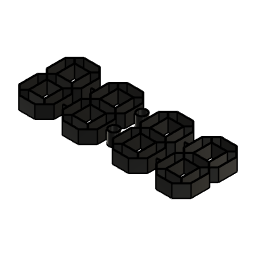
digitalclock_7segment_grid (Autodesk Fusion 360 design; units mm, degrees)
part number: Konfiguration 1
Autodesk Fusion 360 part; units mm, degrees
sketch "Skizze1" plane through (0, 0, 0) normal (0, 0, 1) x (1, 0, 0)
  line L0 (43.4571, -32.4142) -> (38.4571, -37.4142)
  line L1 (38.4571, -37.4142) -> (20.4571, -37.4142)
  line L2 (15.4571, -32.4142) -> (20.4571, -27.4142)
  line L3 (20.4571, -37.4142) -> (15.4571, -32.4142)
  line L4 (20.4571, -27.4142) -> (38.4571, -27.4142)
  line L5 (38.4571, -27.4142) -> (43.4571, -32.4142)
  line L6 (-92114.4293, 91329.2603) -> (-92111.6515, 91326.0366)
  line L7 (-92121.2848, 91323.3531) -> (-92114.4293, 91329.2603)
  line L8 (-92111.6515, 91326.0366) -> (-92106.8214, 91308.6967)
  line L9 (-92112.937, 91302.5267) -> (-92116.4546, 91306.0133)
  line L10 (-92116.4546, 91306.0133) -> (-92121.2848, 91323.3531)
  line L11 (-92118.8697, 91314.6832) -> (-92109.2364, 91317.3666) construction
  line L12 (-92106.8214, 91308.6967) -> (-92112.937, 91302.5267)
  line L13 (38.4571, -5) -> (20.4571, -5)
  line L14 (20.4571, 5) -> (38.4571, 5)
  line L15 (43.4571, 0) -> (38.4571, -5)
  line L16 (38.4571, 5) -> (43.4571, 0)
  line L17 (15.4571, 0) -> (20.4571, 5)
  line L18 (20.4571, -5) -> (15.4571, 0)
  line L19 (38.4571, 27.4142) -> (20.4571, 27.4142)
  line L20 (20.4571, 37.4142) -> (38.4571, 37.4142)
  line L21 (43.4571, 32.4142) -> (38.4571, 27.4142)
  line L22 (38.4571, 37.4142) -> (43.4571, 32.4142)
  line L23 (15.4571, 32.4142) -> (20.4571, 37.4142)
  line L24 (20.4571, 27.4142) -> (15.4571, 32.4142)
  line L25 (9.75, -26.7071) -> (9.75, -5.7071)
  line L26 (19.75, -5.7071) -> (19.75, -26.7071)
  line L27 (14.75, -31.7071) -> (9.75, -26.7071)
  line L28 (19.75, -26.7071) -> (14.75, -31.7071)
  line L29 (14.75, -0.7071) -> (19.75, -5.7071)
  line L30 (9.75, -5.7071) -> (14.75, -0.7071)
  line L31 (19.75, 5.7071) -> (14.75, 0.7071)
  line L32 (14.75, 0.7071) -> (9.75, 5.7071)
  line L33 (9.75, 26.7071) -> (14.75, 31.7071)
  line L34 (9.75, 5.7071) -> (9.75, 26.7071)
  line L35 (19.75, 26.7071) -> (19.75, 5.7071)
  line L36 (14.75, 31.7071) -> (19.75, 26.7071)
  line L37 (49.1642, -26.7071) -> (44.1642, -31.7071)
  line L38 (44.1642, -31.7071) -> (39.1642, -26.7071)
  line L39 (39.1642, -5.7071) -> (44.1642, -0.7071)
  line L40 (39.1642, -26.7071) -> (39.1642, -5.7071)
  line L41 (49.1642, -5.7071) -> (49.1642, -26.7071)
  line L42 (44.1642, -0.7071) -> (49.1642, -5.7071)
  line L43 (49.1642, 5.7071) -> (44.1642, 0.7071)
  line L44 (44.1642, 0.7071) -> (39.1642, 5.7071)
  line L45 (39.1642, 26.7071) -> (44.1642, 31.7071)
  line L46 (39.1642, 5.7071) -> (39.1642, 26.7071)
  line L47 (49.1642, 26.7071) -> (49.1642, 5.7071)
  line L48 (44.1642, 31.7071) -> (49.1642, 26.7071)
  line L49 (49.1642, -16.2071) -> (39.1642, -16.2071) construction
  line L50 (29.4571, -37.4142) -> (29.4571, -27.4142) construction
  line L51 (29.4571, -5) -> (29.4571, 5) construction
  line L52 (29.4571, 27.4142) -> (29.4571, 37.4142) construction
  line L53 (49.1642, 16.2071) -> (39.1642, 16.2071) construction
  line L54 (9.75, 16.2071) -> (19.75, 16.2071) construction
  line L55 (19.75, -16.2071) -> (9.75, -16.2071) construction
  line L56 (38.1642, -26.4142) -> (20.75, -26.4142)
  line L57 (20.75, -26.4142) -> (20.75, -6)
  line L58 (20.75, -6) -> (38.1642, -6)
  line L59 (38.1642, -6) -> (38.1642, -26.4142)
  line L60 (38.1642, 6) -> (20.75, 6)
  line L61 (20.75, 6) -> (20.75, 26.4142)
  line L62 (20.75, 26.4142) -> (38.1642, 26.4142)
  line L63 (38.1642, 26.4142) -> (38.1642, 6)
  line L64 (50.1642, 27.1213) -> (38.8713, 38.4142)
  line L65 (38.8713, 38.4142) -> (20.0429, 38.4142)
  line L66 (20.0429, 38.4142) -> (8.75, 27.1213)
  line L67 (8.75, -27.1213) -> (20.0429, -38.4142)
  line L68 (20.0429, -38.4142) -> (38.8713, -38.4142)
  line L69 (38.8713, -38.4142) -> (50.1642, -27.1213)
  line L70 (50.1642, 5.2929) -> (44.8713, 0)
  line L71 (44.8713, 0) -> (50.1642, -5.2929)
  line L72 (8.75, -5.2929) -> (14.0429, 0)
  line L73 (14.0429, 0) -> (8.75, 5.2929)
  line L74 (50.1642, -27.1213) -> (50.1642, -5.2929)
  line L75 (50.1642, 5.2929) -> (50.1642, 27.1213)
  line L76 (8.75, 27.1213) -> (8.75, 5.2929)
  line L77 (8.75, -5.2929) -> (8.75, -27.1213)
  line L78 (1.75, 0) -> (22.5, 0)
  dimension "d8" = 18
  dimension "d9" = 10
  dimension "d10" = 18
  dimension "d24" = 18
  dimension "d25" = 10
  dimension "d26" = 18
  dimension "d33" = 5
  dimension "d34" = 5
  dimension "d35" = 18
  dimension "d36" = 10
  dimension "d37" = 18
  dimension "d38" = 5
  dimension "d39" = 5
  dimension "d40" = 18
  dimension "d41" = 10
  dimension "d42" = 18
  dimension "d43" = 5
  dimension "d44" = 5
  dimension "d45" = 21
  dimension "d46" = 10
  dimension "d47" = 21
  dimension "d48" = 5
  dimension "d49" = 5
  dimension "d50" = 21
  dimension "d51" = 10
  dimension "d52" = 21
  dimension "d53" = 5
  dimension "d54" = 5
  dimension "d55" = 21
  dimension "d56" = 10
  dimension "d57" = 21
  dimension "d58" = 5
  dimension "d59" = 5
  dimension "d60" = 21
  dimension "d61" = 10
  dimension "d62" = 21
  dimension "d63" = 5
  dimension "d64" = 5
  dimension "d65" = 1
  dimension "d66" = 1
  dimension "d68" = 1
  dimension "d69" = 1
  dimension "d70" = 1
  dimension "d71" = 1
  dimension "d72" = 1
  dimension "d73" = 1
  dimension "d74" = 1
  dimension "d75" = 1
  dimension "d76" = 1
  dimension "d77" = 1
  dimension "d78" = 1
  dimension "d79" = 1
  dimension "d80" = 1
  dimension "d81" = 1
  dimension "d82" = 1
  dimension "d83" = 1
  dimension "d84" = 1
  dimension "d85" = 1
  dimension "d86" = 1
  dimension "d87" = 1
  dimension "d88" = 1
  dimension "d89" = 1
  dimension "d90" = 8.75
  constraint horizontal L1
  constraint perpendicular L2 L3
  constraint parallel L1 L4
  constraint perpendicular L0 L5
  constraint perpendicular L6 L7
  constraint parallel L8 L10
  constraint perpendicular L9 L12
  constraint midpoint L11.start L10
  constraint midpoint L11.end L8
  constraint perpendicular L10 L11
  constraint horizontal L13
  constraint perpendicular L17 L18
  constraint parallel L13 L14
  constraint perpendicular L15 L16
  constraint horizontal L19
  constraint perpendicular L23 L24
  constraint parallel L19 L20
  constraint perpendicular L21 L22
  constraint perpendicular L29 L30
  constraint parallel L25 L26
  constraint perpendicular L27 L28
  constraint perpendicular L33 L36
  constraint parallel L34 L35
  constraint perpendicular L31 L32
  constraint perpendicular L39 L42
  constraint parallel L40 L41
  constraint perpendicular L37 L38
  constraint perpendicular L45 L48
  constraint parallel L46 L47
  constraint perpendicular L43 L44
  constraint vertical L41
  constraint midpoint L41 L49.start
  constraint midpoint L40 L49.end
  constraint midpoint L1 L50.start
  constraint midpoint L4 L50.end
  constraint midpoint L13 L51.start
  constraint midpoint L14 L51.end
  constraint midpoint L19 L52.start
  constraint midpoint L20 L52.end
  constraint midpoint L47 L53.start
  constraint midpoint L46 L53.end
  constraint midpoint L34 L54.start
  constraint midpoint L35 L54.end
  constraint perpendicular L35 L54
  constraint midpoint L26 L55.start
  constraint midpoint L25 L55.end
  constraint perpendicular L25 L55
  constraint perpendicular L40 L49
  constraint perpendicular L1 L50
  constraint perpendicular L19 L52
  constraint perpendicular L13 L51
  constraint perpendicular L47 L53
  constraint collinear L0 L37
  constraint collinear L16 L42
  constraint collinear L17 L30
  constraint collinear L3 L27
  constraint collinear L15 L43
  constraint collinear L22 L48
  constraint collinear L18 L32
  constraint collinear L23 L33
  constraint horizontal L56
  constraint vertical L57
  constraint horizontal L58
  constraint vertical L59
  constraint horizontal L60
  constraint vertical L61
  constraint horizontal L62
  constraint vertical L63
  constraint perpendicular L37 L64
  constraint parallel L37 L66
  constraint parallel L41 L76
  constraint vertical L74
  constraint horizontal L68
  constraint horizontal L65
  constraint parallel L0 L69
  constraint coincident L70.start L74
  constraint perpendicular L70 L71
  constraint coincident L72.start L76
  constraint perpendicular L32 L72
  constraint perpendicular L72 L73
  constraint parallel L42 L71
  constraint collinear L74 L75
  constraint collinear L76 L77
  constraint coincident L17.start L78
  measures "d8" distance of L0.end L1.end
  measures "d9" distance of L1 L4
  measures "d10" distance of L2.end L4.end
  measures "d24" distance of L9.end L7.start
  measures "d25" distance of L8 L10
  measures "d26" distance of L6.end L8.end
  measures "d33" distance of L0.start L1
  measures "d34" distance of L2.start L1
  measures "d35" distance of L13.end L13.start
  measures "d36" distance of L13 L14
  measures "d37" distance of L14.end L14.start
  measures "d38" distance of L15.start L13
  measures "d39" distance of L17.start L13
  measures "d40" distance of L19.end L19.start
  measures "d41" distance of L19 L20
  measures "d42" distance of L20.end L20.start
  measures "d43" distance of L21.start L19
  measures "d44" distance of L23.start L19
  measures "d45" distance of L25.end L25.start
  measures "d46" distance of L25 L26
  measures "d47" distance of L26.end L26.start
  measures "d48" distance of L27.start L25
  measures "d49" distance of L29.start L25
  measures "d50" distance of L33.start L32.end
  measures "d51" distance of L34 L35
  measures "d52" distance of L35.start L31.start
  measures "d53" distance of L31.end L34
  measures "d54" distance of L33.end L34
  measures "d55" distance of L39.start L38.end
  measures "d56" distance of L40 L41
  measures "d57" distance of L41.start L37.start
  measures "d58" distance of L37.end L40
  measures "d59" distance of L39.end L40
  measures "d60" distance of L45.start L44.end
  measures "d61" distance of L46 L47
  measures "d62" distance of L47.start L43.start
  measures "d63" distance of L43.end L46
  measures "d64" distance of L45.end L46
  measures "d65" distance of L5 L38
  measures "d66" distance of L15 L39
  measures "d68" distance of L16 L44
  measures "d69" distance of L21 L45
  measures "d70" distance of L40 L59
  measures "d71" distance of L26 L57
  measures "d72" distance of L4 L56
  measures "d73" distance of L13 L58
  measures "d74" distance of L14 L60
  measures "d75" distance of L35 L61
  measures "d76" distance of L46 L63
  measures "d77" distance of L19 L62
  measures "d78" distance of L41 L74
  measures "d79" distance of L25 L76
  measures "d80" distance of L1 L68
  measures "d81" distance of L27 L67
  measures "d82" distance of L48 L64
  measures "d83" distance of L23 L66
  measures "d84" distance of L20 L65
  measures "d85" distance of L0 L69
  measures "d86" distance of L32 L73
  measures "d87" distance of L30 L72
  measures "d88" distance of L42 L71
  measures "d89" distance of L43 L70
  measures "d90" distance of origin L76
extrude "Extrusion1" add sketch "Skizze1" along normal blind 15 contours L64 L65 L66 L67 L68 L69 L70 L71 L72 L73 L74 L75 L76 L77 makes body 1
ref_plane "Arbeitsebene1" through (55, 0, 0) normal (1, 0, 0) x (0, 1, 0)
mirror "Spiegeln2" about plane through (55, 0, 0) normal (1, 0, 0) of bodies 1 makes body 2
mirror "Spiegeln3" about plane through (0, 0, 0) normal (1, 0, 0) of bodies 1 2 makes body 3 at (-14.5143, 32.4142, 0) makes body 4 at (-95.4857, 32.4142, 0)
sketch "Skizze2" plane through (0, 0, 0) normal (0, 0, 1) x (1, 0, 0)
  circle A0 centre (0, -16.5) radius 5
  circle A1 centre (0, 16.5) radius 5
  circle A2 centre (0, 16.5) radius 6
  circle A3 centre (0, -16.5) radius 6
  line L0 (0, 1.75) -> (0, 22.5)
  dimension "d101" = 10
  dimension "d102" = 10
  dimension "d104" = 33
  dimension "d105" = 1
  dimension "d106" = 1
  dimension "d118" = 16.5
  constraint concentric A1 A2
  constraint concentric A0 A3
  constraint coincident A1.centre L0
  constraint coincident A0.centre L0
  measures "d101" diameter of A0
  measures "d102" diameter of A1
  measures "d104" distance of A0.centre A1.centre
  measures "d105" distance of A0 A3
  measures "d106" distance of A1 A2
  measures "d118" distance of origin A1.centre
extrude "Extrusion2" add sketch "Skizze2" along normal blind 15 separate body contours A1 A2 L0 | A1 A2 L0 | A3 makes body 5 at (5.9702, -17.0974, 10) makes body 6 at (5.9702, 15.9026, 10)
sketch "Skizze3" plane through (0, 0, 0) normal (0, 0, 1) x (1, 0, 0)
sketch "Skizze4" plane through (0, 0, 0) normal (0, 0, 1) x (1, 0, 0)
  line L0 (61.8541, 17) -> (-75.6976, 17)
  line L1 (-75.6976, 17) -> (-75.6976, 16)
  line L2 (-75.6976, 16) -> (61.8541, 16)
  line L3 (61.8541, 16) -> (61.8541, 17)
  line L4 (63.4741, -16) -> (-75.6976, -16)
  line L5 (-75.6976, -16) -> (-75.6976, -17)
  line L6 (-75.6976, -17) -> (63.4741, -17)
  line L7 (63.4741, -17) -> (63.4741, -16)
  circle A0 centre (0, 16.5) radius 5
  circle A1 centre (0, -16.5) radius 5
  line L8 (8.75, 27.1213) -> (8.75, 5.2929)
  line L9 (38.4571, -27.4142) -> (20.4571, -27.4142)
  line L10 (20.4571, -27.4142) -> (15.4571, -32.4142)
  line L11 (15.4571, -32.4142) -> (20.4571, -37.4142)
  line L12 (20.4571, -37.4142) -> (38.4571, -37.4142)
  line L13 (38.4571, -37.4142) -> (43.4571, -32.4142)
  line L14 (43.4571, -32.4142) -> (38.4571, -27.4142)
  line L15 (44.1642, 31.7071) -> (39.1642, 26.7071)
  line L16 (39.1642, 26.7071) -> (39.1642, 5.7071)
  line L17 (39.1642, 5.7071) -> (44.1642, 0.7071)
  line L18 (44.1642, 0.7071) -> (49.1642, 5.7071)
  line L19 (49.1642, 5.7071) -> (49.1642, 26.7071)
  line L20 (49.1642, 26.7071) -> (44.1642, 31.7071)
  line L21 (14.75, 31.7071) -> (9.75, 26.7071)
  line L22 (9.75, 26.7071) -> (9.75, 5.7071)
  line L23 (9.75, 5.7071) -> (14.75, 0.7071)
  line L24 (14.75, 0.7071) -> (19.75, 5.7071)
  line L25 (19.75, 5.7071) -> (19.75, 26.7071)
  line L26 (19.75, 26.7071) -> (14.75, 31.7071)
  line L27 (20.4571, 27.4142) -> (38.4571, 27.4142)
  line L28 (38.4571, 27.4142) -> (43.4571, 32.4142)
  line L29 (43.4571, 32.4142) -> (38.4571, 37.4142)
  line L30 (38.4571, 37.4142) -> (20.4571, 37.4142)
  line L31 (20.4571, 37.4142) -> (15.4571, 32.4142)
  line L32 (15.4571, 32.4142) -> (20.4571, 27.4142)
  line L33 (38.1642, 26.4142) -> (20.75, 26.4142)
  line L34 (20.75, 26.4142) -> (20.75, 6)
  line L35 (20.75, 6) -> (38.1642, 6)
  line L36 (38.1642, 6) -> (38.1642, 26.4142)
  line L37 (44.1642, -0.7071) -> (39.1642, -5.7071)
  line L38 (39.1642, -5.7071) -> (39.1642, -26.7071)
  line L39 (39.1642, -26.7071) -> (44.1642, -31.7071)
  line L40 (44.1642, -31.7071) -> (49.1642, -26.7071)
  line L41 (49.1642, -26.7071) -> (49.1642, -5.7071)
  line L42 (49.1642, -5.7071) -> (44.1642, -0.7071)
  line L43 (20.4571, -5) -> (38.4571, -5)
  line L44 (38.4571, -5) -> (43.4571, 0)
  line L45 (43.4571, 0) -> (38.4571, 5)
  line L46 (38.4571, 5) -> (20.4571, 5)
  line L47 (20.4571, 5) -> (15.4571, 0)
  line L48 (15.4571, 0) -> (20.4571, -5)
  line L49 (9.75, -5.7071) -> (9.75, -26.7071)
  line L50 (9.75, -26.7071) -> (14.75, -31.7071)
  line L51 (14.75, -31.7071) -> (19.75, -26.7071)
  line L52 (19.75, -26.7071) -> (19.75, -5.7071)
  line L53 (19.75, -5.7071) -> (14.75, -0.7071)
  line L54 (14.75, -0.7071) -> (9.75, -5.7071)
  line L55 (38.1642, -6) -> (20.75, -6)
  line L56 (20.75, -6) -> (20.75, -26.4142)
  line L57 (20.75, -26.4142) -> (38.1642, -26.4142)
  line L58 (38.1642, -26.4142) -> (38.1642, -6)
  line L59 (8.75, -5.2929) -> (14.0429, 0)
  line L60 (14.0429, 0) -> (8.75, 5.2929)
  line L61 (8.75, 5.2929) -> (8.75, 27.1213)
  line L62 (8.75, 27.1213) -> (20.0429, 38.4142)
  line L63 (20.0429, 38.4142) -> (38.8713, 38.4142)
  line L64 (38.8713, 38.4142) -> (50.1642, 27.1213)
  line L65 (50.1642, 27.1213) -> (50.1642, 5.2929)
  line L66 (50.1642, 5.2929) -> (44.8713, 0)
  line L67 (44.8713, 0) -> (50.1642, -5.2929)
  line L68 (50.1642, -5.2929) -> (50.1642, -27.1213)
  line L69 (50.1642, -27.1213) -> (38.8713, -38.4142)
  line L70 (38.8713, -38.4142) -> (20.0429, -38.4142)
  line L71 (20.0429, -38.4142) -> (8.75, -27.1213)
  line L72 (8.75, -27.1213) -> (8.75, -5.2929)
  line L73 (89.5429, -27.4142) -> (71.5429, -27.4142)
  line L74 (71.5429, -27.4142) -> (66.5429, -32.4142)
  line L75 (66.5429, -32.4142) -> (71.5429, -37.4142)
  line L76 (71.5429, -37.4142) -> (89.5429, -37.4142)
  line L77 (89.5429, -37.4142) -> (94.5429, -32.4142)
  line L78 (94.5429, -32.4142) -> (89.5429, -27.4142)
  line L79 (70.8358, 26.7071) -> (65.8358, 31.7071)
  line L80 (65.8358, 31.7071) -> (60.8358, 26.7071)
  line L81 (60.8358, 26.7071) -> (60.8358, 5.7071)
  line L82 (60.8358, 5.7071) -> (65.8358, 0.7071)
  line L83 (65.8358, 0.7071) -> (70.8358, 5.7071)
  line L84 (70.8358, 5.7071) -> (70.8358, 26.7071)
  line L85 (100.25, 26.7071) -> (95.25, 31.7071)
  line L86 (95.25, 31.7071) -> (90.25, 26.7071)
  line L87 (90.25, 26.7071) -> (90.25, 5.7071)
  line L88 (90.25, 5.7071) -> (95.25, 0.7071)
  line L89 (95.25, 0.7071) -> (100.25, 5.7071)
  line L90 (100.25, 5.7071) -> (100.25, 26.7071)
  line L91 (71.5429, 27.4142) -> (89.5429, 27.4142)
  line L92 (89.5429, 27.4142) -> (94.5429, 32.4142)
  line L93 (94.5429, 32.4142) -> (89.5429, 37.4142)
  line L94 (89.5429, 37.4142) -> (71.5429, 37.4142)
  line L95 (71.5429, 37.4142) -> (66.5429, 32.4142)
  line L96 (66.5429, 32.4142) -> (71.5429, 27.4142)
  line L97 (89.25, 26.4142) -> (71.8358, 26.4142)
  line L98 (71.8358, 26.4142) -> (71.8358, 6)
  line L99 (71.8358, 6) -> (89.25, 6)
  line L100 (89.25, 6) -> (89.25, 26.4142)
  line L101 (70.8358, -5.7071) -> (65.8358, -0.7071)
  line L102 (65.8358, -0.7071) -> (60.8358, -5.7071)
  line L103 (60.8358, -5.7071) -> (60.8358, -26.7071)
  line L104 (60.8358, -26.7071) -> (65.8358, -31.7071)
  line L105 (65.8358, -31.7071) -> (70.8358, -26.7071)
  line L106 (70.8358, -26.7071) -> (70.8358, -5.7071)
  line L107 (71.5429, -5) -> (89.5429, -5)
  line L108 (89.5429, -5) -> (94.5429, 0)
  line L109 (94.5429, 0) -> (89.5429, 5)
  line L110 (89.5429, 5) -> (71.5429, 5)
  line L111 (71.5429, 5) -> (66.5429, 0)
  line L112 (66.5429, 0) -> (71.5429, -5)
  line L113 (100.25, -26.7071) -> (100.25, -5.7071)
  line L114 (100.25, -5.7071) -> (95.25, -0.7071)
  line L115 (95.25, -0.7071) -> (90.25, -5.7071)
  line L116 (90.25, -5.7071) -> (90.25, -26.7071)
  line L117 (90.25, -26.7071) -> (95.25, -31.7071)
  line L118 (95.25, -31.7071) -> (100.25, -26.7071)
  line L119 (89.25, -6) -> (71.8358, -6)
  line L120 (71.8358, -6) -> (71.8358, -26.4142)
  line L121 (71.8358, -26.4142) -> (89.25, -26.4142)
  line L122 (89.25, -26.4142) -> (89.25, -6)
  line L123 (95.9571, 0) -> (101.25, -5.2929)
  line L124 (101.25, -5.2929) -> (101.25, -27.1213)
  line L125 (101.25, -27.1213) -> (89.9571, -38.4142)
  line L126 (89.9571, -38.4142) -> (71.1287, -38.4142)
  line L127 (71.1287, -38.4142) -> (59.8358, -27.1213)
  line L128 (59.8358, -27.1213) -> (59.8358, -5.2929)
  line L129 (59.8358, -5.2929) -> (65.1287, 0)
  line L130 (65.1287, 0) -> (59.8358, 5.2929)
  line L131 (59.8358, 5.2929) -> (59.8358, 27.1213)
  line L132 (59.8358, 27.1213) -> (71.1287, 38.4142)
  line L133 (71.1287, 38.4142) -> (89.9571, 38.4142)
  line L134 (89.9571, 38.4142) -> (101.25, 27.1213)
  line L135 (101.25, 27.1213) -> (101.25, 5.2929)
  line L136 (101.25, 5.2929) -> (95.9571, 0)
  line L137 (-20.4571, -27.4142) -> (-38.4571, -27.4142)
  line L138 (-38.4571, -27.4142) -> (-43.4571, -32.4142)
  line L139 (-43.4571, -32.4142) -> (-38.4571, -37.4142)
  line L140 (-38.4571, -37.4142) -> (-20.4571, -37.4142)
  line L141 (-20.4571, -37.4142) -> (-15.4571, -32.4142)
  line L142 (-15.4571, -32.4142) -> (-20.4571, -27.4142)
  line L143 (-39.1642, 26.7071) -> (-44.1642, 31.7071)
  line L144 (-44.1642, 31.7071) -> (-49.1642, 26.7071)
  line L145 (-49.1642, 26.7071) -> (-49.1642, 5.7071)
  line L146 (-49.1642, 5.7071) -> (-44.1642, 0.7071)
  line L147 (-44.1642, 0.7071) -> (-39.1642, 5.7071)
  line L148 (-39.1642, 5.7071) -> (-39.1642, 26.7071)
  line L149 (-9.75, 26.7071) -> (-14.75, 31.7071)
  line L150 (-14.75, 31.7071) -> (-19.75, 26.7071)
  line L151 (-19.75, 26.7071) -> (-19.75, 5.7071)
  line L152 (-19.75, 5.7071) -> (-14.75, 0.7071)
  line L153 (-14.75, 0.7071) -> (-9.75, 5.7071)
  line L154 (-9.75, 5.7071) -> (-9.75, 26.7071)
  line L155 (-38.4571, 27.4142) -> (-20.4571, 27.4142)
  line L156 (-20.4571, 27.4142) -> (-15.4571, 32.4142)
  line L157 (-15.4571, 32.4142) -> (-20.4571, 37.4142)
  line L158 (-20.4571, 37.4142) -> (-38.4571, 37.4142)
  line L159 (-38.4571, 37.4142) -> (-43.4571, 32.4142)
  line L160 (-43.4571, 32.4142) -> (-38.4571, 27.4142)
  line L161 (-20.75, 26.4142) -> (-38.1642, 26.4142)
  line L162 (-38.1642, 26.4142) -> (-38.1642, 6)
  line L163 (-38.1642, 6) -> (-20.75, 6)
  line L164 (-20.75, 6) -> (-20.75, 26.4142)
  line L165 (-39.1642, -5.7071) -> (-44.1642, -0.7071)
  line L166 (-44.1642, -0.7071) -> (-49.1642, -5.7071)
  line L167 (-49.1642, -5.7071) -> (-49.1642, -26.7071)
  line L168 (-49.1642, -26.7071) -> (-44.1642, -31.7071)
  line L169 (-44.1642, -31.7071) -> (-39.1642, -26.7071)
  line L170 (-39.1642, -26.7071) -> (-39.1642, -5.7071)
  line L171 (-38.4571, -5) -> (-20.4571, -5)
  line L172 (-20.4571, -5) -> (-15.4571, 0)
  line L173 (-15.4571, 0) -> (-20.4571, 5)
  line L174 (-20.4571, 5) -> (-38.4571, 5)
  line L175 (-38.4571, 5) -> (-43.4571, 0)
  line L176 (-43.4571, 0) -> (-38.4571, -5)
  line L177 (-9.75, -26.7071) -> (-9.75, -5.7071)
  line L178 (-9.75, -5.7071) -> (-14.75, -0.7071)
  line L179 (-14.75, -0.7071) -> (-19.75, -5.7071)
  line L180 (-19.75, -5.7071) -> (-19.75, -26.7071)
  line L181 (-19.75, -26.7071) -> (-14.75, -31.7071)
  line L182 (-14.75, -31.7071) -> (-9.75, -26.7071)
  line L183 (-20.75, -6) -> (-38.1642, -6)
  line L184 (-38.1642, -6) -> (-38.1642, -26.4142)
  line L185 (-38.1642, -26.4142) -> (-20.75, -26.4142)
  line L186 (-20.75, -26.4142) -> (-20.75, -6)
  line L187 (-14.0429, 0) -> (-8.75, -5.2929)
  line L188 (-8.75, -5.2929) -> (-8.75, -27.1213)
  line L189 (-8.75, -27.1213) -> (-20.0429, -38.4142)
  line L190 (-20.0429, -38.4142) -> (-38.8713, -38.4142)
  line L191 (-38.8713, -38.4142) -> (-50.1642, -27.1213)
  line L192 (-50.1642, -27.1213) -> (-50.1642, -5.2929)
  line L193 (-50.1642, -5.2929) -> (-44.8713, 0)
  line L194 (-44.8713, 0) -> (-50.1642, 5.2929)
  line L195 (-50.1642, 5.2929) -> (-50.1642, 27.1213)
  line L196 (-50.1642, 27.1213) -> (-38.8713, 38.4142)
  line L197 (-38.8713, 38.4142) -> (-20.0429, 38.4142)
  line L198 (-20.0429, 38.4142) -> (-8.75, 27.1213)
  line L199 (-8.75, 27.1213) -> (-8.75, 5.2929)
  line L200 (-8.75, 5.2929) -> (-14.0429, 0)
  line L201 (-71.5429, -27.4142) -> (-89.5429, -27.4142)
  line L202 (-89.5429, -27.4142) -> (-94.5429, -32.4142)
  line L203 (-94.5429, -32.4142) -> (-89.5429, -37.4142)
  line L204 (-89.5429, -37.4142) -> (-71.5429, -37.4142)
  line L205 (-71.5429, -37.4142) -> (-66.5429, -32.4142)
  line L206 (-66.5429, -32.4142) -> (-71.5429, -27.4142)
  line L207 (-65.8358, 31.7071) -> (-70.8358, 26.7071)
  line L208 (-70.8358, 26.7071) -> (-70.8358, 5.7071)
  line L209 (-70.8358, 5.7071) -> (-65.8358, 0.7071)
  line L210 (-65.8358, 0.7071) -> (-60.8358, 5.7071)
  line L211 (-60.8358, 5.7071) -> (-60.8358, 26.7071)
  line L212 (-60.8358, 26.7071) -> (-65.8358, 31.7071)
  line L213 (-95.25, 31.7071) -> (-100.25, 26.7071)
  line L214 (-100.25, 26.7071) -> (-100.25, 5.7071)
  line L215 (-100.25, 5.7071) -> (-95.25, 0.7071)
  line L216 (-95.25, 0.7071) -> (-90.25, 5.7071)
  line L217 (-90.25, 5.7071) -> (-90.25, 26.7071)
  line L218 (-90.25, 26.7071) -> (-95.25, 31.7071)
  line L219 (-89.5429, 27.4142) -> (-71.5429, 27.4142)
  line L220 (-71.5429, 27.4142) -> (-66.5429, 32.4142)
  line L221 (-66.5429, 32.4142) -> (-71.5429, 37.4142)
  line L222 (-71.5429, 37.4142) -> (-89.5429, 37.4142)
  line L223 (-89.5429, 37.4142) -> (-94.5429, 32.4142)
  line L224 (-94.5429, 32.4142) -> (-89.5429, 27.4142)
  line L225 (-71.8358, 26.4142) -> (-89.25, 26.4142)
  line L226 (-89.25, 26.4142) -> (-89.25, 6)
  line L227 (-89.25, 6) -> (-71.8358, 6)
  line L228 (-71.8358, 6) -> (-71.8358, 26.4142)
  line L229 (-65.8358, -0.7071) -> (-70.8358, -5.7071)
  line L230 (-70.8358, -5.7071) -> (-70.8358, -26.7071)
  line L231 (-70.8358, -26.7071) -> (-65.8358, -31.7071)
  line L232 (-65.8358, -31.7071) -> (-60.8358, -26.7071)
  line L233 (-60.8358, -26.7071) -> (-60.8358, -5.7071)
  line L234 (-60.8358, -5.7071) -> (-65.8358, -0.7071)
  line L235 (-89.5429, -5) -> (-71.5429, -5)
  line L236 (-71.5429, -5) -> (-66.5429, 0)
  line L237 (-66.5429, 0) -> (-71.5429, 5)
  line L238 (-71.5429, 5) -> (-89.5429, 5)
  line L239 (-89.5429, 5) -> (-94.5429, 0)
  line L240 (-94.5429, 0) -> (-89.5429, -5)
  line L241 (-100.25, -5.7071) -> (-100.25, -26.7071)
  line L242 (-100.25, -26.7071) -> (-95.25, -31.7071)
  line L243 (-95.25, -31.7071) -> (-90.25, -26.7071)
  line L244 (-90.25, -26.7071) -> (-90.25, -5.7071)
  line L245 (-90.25, -5.7071) -> (-95.25, -0.7071)
  line L246 (-95.25, -0.7071) -> (-100.25, -5.7071)
  line L247 (-71.8358, -6) -> (-89.25, -6)
  line L248 (-89.25, -6) -> (-89.25, -26.4142)
  line L249 (-89.25, -26.4142) -> (-71.8358, -26.4142)
  line L250 (-71.8358, -26.4142) -> (-71.8358, -6)
  line L251 (-101.25, -5.2929) -> (-95.9571, 0)
  line L252 (-95.9571, 0) -> (-101.25, 5.2929)
  line L253 (-101.25, 5.2929) -> (-101.25, 27.1213)
  line L254 (-101.25, 27.1213) -> (-89.9571, 38.4142)
  line L255 (-89.9571, 38.4142) -> (-71.1287, 38.4142)
  line L256 (-71.1287, 38.4142) -> (-59.8358, 27.1213)
  line L257 (-59.8358, 27.1213) -> (-59.8358, 5.2929)
  line L258 (-59.8358, 5.2929) -> (-65.1287, 0)
  line L259 (-65.1287, 0) -> (-59.8358, -5.2929)
  line L260 (-59.8358, -5.2929) -> (-59.8358, -27.1213)
  line L261 (-59.8358, -27.1213) -> (-71.1287, -38.4142)
  line L262 (-71.1287, -38.4142) -> (-89.9571, -38.4142)
  line L263 (-89.9571, -38.4142) -> (-101.25, -27.1213)
  line L264 (-101.25, -27.1213) -> (-101.25, -5.2929)
  dimension "d109" = 1
  dimension "d110" = 1
  dimension "d112" = 0.5
  dimension "d113" = 0.5
  constraint horizontal L0
  constraint vertical L1
  constraint horizontal L2
  constraint vertical L3
  constraint horizontal L4
  constraint vertical L5
  constraint horizontal L6
  constraint vertical L7
  measures "d109" distance of L0 L2
  measures "d110" distance of L4 L6
  measures "d112" distance of L0 A0.centre
  measures "d113" distance of L4 A1.centre
extrude "Extrusion3" add sketch "Skizze4" along normal blind 10 contours L0 L2 L65 L131 | L4 L6 L68 L128 | L0 L2 A0 L8 L61 | L0 L2 A0 L199 | L4 L6 A1 L72 | L4 L6 A1 L188 | L0 L2 L195 L257 | L4 L6 L192 L260 bodies 1 5 2 3 4 6
sketch "Skizze5" plane through (0, 0, 0) normal (0, 0, 1) x (1, 0, 0)
  circle A0 centre (0, 0) radius 2
  circle A1 centre (-29.5, -33) radius 2
  circle A2 centre (-44.25, -16.5) radius 2
  circle A3 centre (-29.5, -16.5) radius 2
  circle A4 centre (-14.75, -16.5) radius 2
  circle A5 centre (-29.5, 0) radius 2
  circle A6 centre (-44.25, 16.5) radius 2
  circle A7 centre (-29.5, 16.5) radius 2
  circle A8 centre (-14.75, 16.5) radius 2
  circle A9 centre (0, -33) radius 2
  circle A10 centre (29.5, -33) radius 2
  circle A11 centre (0, -16.5) radius 2
  circle A12 centre (14.75, -16.5) radius 2
  circle A13 centre (29.5, -16.5) radius 2
  circle A14 centre (44.25, -16.5) radius 2
  circle A15 centre (29.5, 0) radius 2
  circle A16 centre (0, 16.5) radius 2
  circle A17 centre (14.75, 16.5) radius 2
  circle A18 centre (29.5, 16.5) radius 2
  circle A19 centre (44.25, 16.5) radius 2
  circle A20 centre (-29.5, 33) radius 2
  circle A21 centre (0, 33) radius 2
  circle A22 centre (29.5, 33) radius 2
  line L0 (55, 0.4199) -> (55, 12.1783)
  circle A23 centre (65.75, 16.5) radius 2
  circle A24 centre (65.75, -16.5) radius 2
  circle A25 centre (80.5, -33) radius 2
  circle A26 centre (95.25, -16.5) radius 2
  circle A27 centre (80.5, -16.5) radius 2
  circle A28 centre (80.5, 0) radius 2
  circle A29 centre (95.25, 16.5) radius 2
  circle A30 centre (80.5, 16.5) radius 2
  circle A31 centre (80.5, 33) radius 2
  line L1 (0, 2.5) -> (0, 20)
  circle A32 centre (-80.5, 33) radius 2
  circle A33 centre (-65.75, 16.5) radius 2
  circle A34 centre (-80.5, 16.5) radius 2
  circle A35 centre (-95.25, 16.5) radius 2
  circle A36 centre (-80.5, 0) radius 2
  circle A37 centre (-65.75, -16.5) radius 2
  circle A38 centre (-80.5, -16.5) radius 2
  circle A39 centre (-95.25, -16.5) radius 2
  circle A40 centre (-80.5, -33) radius 2
  circle A41 centre (0, 0) radius 110
  circle A42 centre (0, -49.5) radius 2
  circle A43 centre (14.75, -49.5) radius 2
  circle A44 centre (29.5, -49.5) radius 2
  circle A45 centre (44.25, -49.5) radius 2
  circle A46 centre (65.75, -49.5) radius 2
  circle A47 centre (80.5, -49.5) radius 2
  circle A48 centre (95.25, -49.5) radius 2
  circle A49 centre (-14.75, -49.5) radius 2
  circle A50 centre (-29.5, -49.5) radius 2
  circle A51 centre (-44.25, -49.5) radius 2
  circle A52 centre (-65.75, -49.5) radius 2
  circle A53 centre (-80.5, -49.5) radius 2
  circle A54 centre (-95.25, -49.5) radius 2
  circle A55 centre (0, -66) radius 2
  circle A56 centre (29.5, -66) radius 2
  circle A57 centre (80.5, -66) radius 2
  circle A58 centre (-29.5, -66) radius 2
  circle A59 centre (-80.5, -66) radius 2
  circle A60 centre (0, -82.5) radius 2
  circle A61 centre (14.75, -82.5) radius 2
  circle A62 centre (29.5, -82.5) radius 2
  circle A63 centre (44.25, -82.5) radius 2
  circle A64 centre (65.75, -82.5) radius 2
  circle A65 centre (-14.75, -82.5) radius 2
  circle A66 centre (-29.5, -82.5) radius 2
  circle A67 centre (-44.25, -82.5) radius 2
  circle A68 centre (-65.75, -82.5) radius 2
  circle A69 centre (0, -99) radius 2
  circle A70 centre (29.5, -99) radius 2
  circle A71 centre (-29.5, -99) radius 2
  circle A72 centre (95.25, 49.5) radius 2
  circle A73 centre (80.5, 49.5) radius 2
  circle A74 centre (65.75, 49.5) radius 2
  circle A75 centre (44.25, 49.5) radius 2
  circle A76 centre (29.5, 49.5) radius 2
  circle A77 centre (14.75, 49.5) radius 2
  circle A78 centre (0, 49.5) radius 2
  circle A79 centre (-14.75, 49.5) radius 2
  circle A80 centre (-29.5, 49.5) radius 2
  circle A81 centre (-44.25, 49.5) radius 2
  circle A82 centre (-65.75, 49.5) radius 2
  circle A83 centre (-80.5, 49.5) radius 2
  circle A84 centre (-95.25, 49.5) radius 2
  circle A85 centre (80.5, 66) radius 2
  circle A86 centre (29.5, 66) radius 2
  circle A87 centre (0, 66) radius 2
  circle A88 centre (-29.5, 66) radius 2
  circle A89 centre (-80.5, 66) radius 2
  circle A90 centre (65.75, 82.5) radius 2
  circle A91 centre (44.25, 82.5) radius 2
  circle A92 centre (29.5, 82.5) radius 2
  circle A93 centre (14.75, 82.5) radius 2
  circle A94 centre (0, 82.5) radius 2
  circle A95 centre (-14.75, 82.5) radius 2
  circle A96 centre (-29.5, 82.5) radius 2
  circle A97 centre (-44.25, 82.5) radius 2
  circle A98 centre (-65.75, 82.5) radius 2
  circle A99 centre (29.5, 99) radius 2
  circle A100 centre (0, 99) radius 2
  circle A101 centre (-29.5, 99) radius 2
  dimension "d116" = 4
  dimension "d125" = 220
  constraint coincident A0.centre A41.centre
  constraint symmetric A10 L0 A25
  constraint symmetric A12 L0 A26
  constraint symmetric A13 L0 A27
  constraint symmetric A14 L0 A24
  constraint symmetric A15 L0 A28
  constraint symmetric A17 L0 A29
  constraint symmetric A18 L0 A30
  constraint symmetric A19 L0 A23
  constraint symmetric A22 L0 A31
  constraint symmetric A23 L1 A33
  constraint symmetric A24 L1 A37
  constraint symmetric A25 L1 A40
  constraint symmetric A26 L1 A39
  constraint symmetric A27 L1 A38
  constraint symmetric A28 L1 A36
  constraint symmetric A29 L1 A35
  constraint symmetric A30 L1 A34
  constraint symmetric A31 L1 A32
  measures "d116" diameter of A0
  measures "d125" diameter of A41
equation "segment_length_hori = 18 mm"
equation "segment_width = 10 mm"
equation "wall_width = 1 mm"
equation "d8 = segment_length_hori"
equation "d9 = segment_width"
equation "d10 = segment_length_hori"
equation "d24 = segment_length_hori"
equation "d25 = segment_width"
equation "d26 = segment_length_hori"
equation "d33 = segment_width / 2"
equation "d34 = segment_width / 2"
equation "d35 = segment_length_hori"
equation "d36 = segment_width"
equation "d37 = segment_length_hori"
equation "d38 = segment_width / 2"
equation "d39 = segment_width / 2"
equation "d40 = segment_length_hori"
equation "d41 = segment_width"
equation "d42 = segment_length_hori"
equation "d43 = segment_width / 2"
equation "d44 = segment_width / 2"
equation "d45 = segment_length_vertical"
equation "d46 = segment_width"
equation "d47 = segment_length_vertical"
equation "d48 = segment_width / 2"
equation "d49 = segment_width / 2"
equation "d50 = segment_length_vertical"
equation "d51 = segment_width"
equation "d52 = segment_length_vertical"
equation "d53 = segment_width / 2"
equation "d54 = segment_width / 2"
equation "d55 = segment_length_vertical"
equation "d56 = segment_width"
equation "d57 = segment_length_vertical"
equation "d58 = segment_width / 2"
equation "d59 = segment_width / 2"
equation "d60 = segment_length_vertical"
equation "d61 = segment_width"
equation "d62 = segment_length_vertical"
equation "d63 = segment_width / 2"
equation "d64 = segment_width / 2"
equation "d65 = wall_width"
equation "d66 = wall_width"
equation "d68 = wall_width"
equation "d69 = wall_width"
equation "d70 = wall_width"
equation "d71 = wall_width"
equation "d72 = wall_width"
equation "d73 = wall_width"
equation "d74 = wall_width"
equation "d75 = wall_width"
equation "d76 = wall_width"
equation "d77 = wall_width"
equation "d78 = wall_width"
equation "d79 = wall_width"
equation "d80 = wall_width"
equation "d81 = wall_width"
equation "d82 = wall_width"
equation "d83 = wall_width"
equation "d84 = wall_width"
equation "d85 = wall_width"
equation "d86 = wall_width"
equation "d87 = wall_width"
equation "d88 = wall_width"
equation "d89 = wall_width"
equation "d104 = ( 2 * 16.5 ) * 1 mm"
equation "d105 = wall_width"
equation "d106 = wall_width"
equation "d109 = wall_width"
equation "d110 = wall_width"
equation "d112 = wall_width / 2"
equation "d113 = wall_width / 2"
equation "segment_length_vertical = 21 mm"
